Autodesk Fusion 360 part; units mm, degrees
(part 5 of 6)
  spline S167 degree 3 poles (6.8323, 73.9658) (7.1559, 73.6374) (7.8437, 72.9395) (8.0667, 71.9824) (8.1848, 71.4756) knots 0 0 0 0 0.135648 0.28832 0.28832 0.28832 0.28832
  line L106 (11.9153, 74.5713) -> (11.9153, 64.2002)
  line L107 (11.9153, 64.2002) -> (10.1575, 64.2002)
  line L108 (10.1575, 64.2002) -> (10.1575, 74.5713)
  line L109 (10.1575, 74.5713) -> (11.9153, 74.5713)
  line L110 (18.6047, 74.5713) -> (18.6047, 64.2002)
  line L111 (18.6047, 64.2002) -> (17.0227, 64.2002)
  line L112 (17.0227, 64.2002) -> (17.0227, 65.7724)
  spline S168 degree 3 poles (17.0227, 65.7724) (16.8465, 65.453) (16.5467, 64.9096) (16.0919, 64.4902) (15.9045, 64.3174) knots 0 0 0 0 0.1085 0.184546 0.184546 0.184546 0.184546
  spline S169 degree 3 poles (15.9045, 64.3174) (15.7296, 64.2148) (15.3808, 64.0103) (14.9776, 63.9806) (14.7766, 63.9658) knots 0 0 0 0 0.059943 0.119555 0.119555 0.119555 0.119555
  spline S170 degree 3 poles (14.7766, 63.9658) (14.4721, 63.9939) (13.8303, 64.053) (13.2663, 64.3671) (12.97, 64.5322) knots 0 0 0 0 0.090712 0.191197 0.191197 0.191197 0.191197
  line L113 (12.97, 64.5322) -> (13.5754, 66.1631)
  spline S171 degree 3 poles (13.5754, 66.1631) (13.7857, 66.052) (14.1903, 65.8384) (14.6457, 65.8004) (14.8645, 65.7822) knots 0 0 0 0 0.070499 0.135652 0.135652 0.135652 0.135652
  spline S172 degree 3 poles (14.8645, 65.7822) (15.0516, 65.7966) (15.4257, 65.8254) (15.7417, 66.0278) (15.8996, 66.1289) knots 0 0 0 0 0.05537 0.110689 0.110689 0.110689 0.110689
  spline S173 degree 3 poles (15.8996, 66.1289) (16.0426, 66.2586) (16.3376, 66.5264) (16.4803, 66.8988) (16.5539, 67.0908) knots 0 0 0 0 0.057074 0.117791 0.117791 0.117791 0.117791
  spline S174 degree 3 poles (16.5539, 67.0908) (16.6394, 67.4162) (16.8158, 68.0883) (16.8363, 68.7831) (16.8469, 69.1416) knots 0 0 0 0 0.100574 0.207758 0.207758 0.207758 0.207758
  line L114 (16.8469, 69.1416) -> (16.8469, 74.5713)
  line L115 (16.8469, 74.5713) -> (18.6047, 74.5713)
  line L116 (40.3918, 71.2314) -> (38.5754, 71.456)
  spline S175 degree 3 poles (38.5754, 71.456) (38.7423, 71.9516) (39.0652, 72.9106) (39.8082, 73.5957) (40.1672, 73.9267) knots 0 0 0 0 0.154068 0.298151 0.298151 0.298151 0.298151
  spline S176 degree 3 poles (40.1672, 73.9267) (40.5971, 74.1828) (41.5099, 74.7266) (42.5734, 74.7783) (43.136, 74.8056) knots 0 0 0 0 0.147834 0.313845 0.313845 0.313845 0.313845
  spline S177 degree 3 poles (43.136, 74.8056) (43.8438, 74.7587) (45.1975, 74.669) (46.2447, 73.8128) (46.7444, 73.4043) knots 0 0 0 0 0.206966 0.395783 0.395783 0.395783 0.395783
  spline S178 degree 3 poles (46.7444, 73.4043) (47.1326, 72.8627) (47.9713, 71.6927) (48.0403, 70.249) (48.0774, 69.4736) knots 0 0 0 0 0.195785 0.422974 0.422974 0.422974 0.422974
  spline S179 degree 3 poles (48.0774, 69.4736) (48.0408, 68.6725) (47.973, 67.1854) (47.1222, 65.9712) (46.7297, 65.4111) knots 0 0 0 0 0.234851 0.435929 0.435929 0.435929 0.435929
  spline S180 degree 3 poles (46.7297, 65.4111) (46.239, 64.9896) (45.2337, 64.1262) (43.9108, 64.0201) (43.2336, 63.9658) knots 0 0 0 0 0.188967 0.387114 0.387114 0.387114 0.387114
  spline S181 degree 3 poles (43.2336, 63.9658) (42.5767, 64.0198) (41.2894, 64.1256) (40.3132, 64.9688) (39.8352, 65.3818) knots 0 0 0 0 0.192252 0.37676 0.37676 0.37676 0.37676
  spline S182 degree 3 poles (39.8352, 65.3818) (39.4513, 65.931) (38.6184, 67.1223) (38.5524, 68.5803) (38.5168, 69.3662) knots 0 0 0 0 0.197018 0.427415 0.427415 0.427415 0.427415
  spline S183 degree 3 poles (38.5168, 69.3662) (38.5175, 69.4313) (38.5189, 69.5876) (38.5238, 69.7438) (38.5266, 69.8349) knots 0 0 0 0 0.019533 0.046886 0.046886 0.046886 0.046886
  line L117 (38.5266, 69.8349) -> (46.261, 69.8349)
  spline S184 degree 3 poles (46.261, 69.8349) (46.2102, 70.3557) (46.1165, 71.3165) (45.5525, 72.0954) (45.2942, 72.4521) knots 0 0 0 0 0.153651 0.283492 0.283492 0.283492 0.283492
  spline S185 degree 3 poles (45.2942, 72.4521) (44.9846, 72.717) (44.3597, 73.2517) (43.5399, 73.3239) (43.1262, 73.3603) knots 0 0 0 0 0.119065 0.24035 0.24035 0.24035 0.24035
  spline S186 degree 3 poles (43.1262, 73.3603) (42.8199, 73.3422) (42.2277, 73.3072) (41.7207, 73.0006) (41.4758, 72.8525) knots 0 0 0 0 0.090495 0.175003 0.175003 0.175003 0.175003
  spline S187 degree 3 poles (41.4758, 72.8525) (41.255, 72.6441) (40.7715, 72.1877) (40.5255, 71.5681) (40.3918, 71.2314) knots 0 0 0 0 0.090002 0.197114 0.197114 0.197114 0.197114
  line L118 (64.1711, 74.5713) -> (64.1711, 64.2002)
  line L119 (64.1711, 64.2002) -> (62.5891, 64.2002)
  line L120 (62.5891, 64.2002) -> (62.5891, 65.6748)
  spline S188 degree 3 poles (62.5891, 65.6748) (62.1608, 65.1763) (61.2915, 64.1647) (59.9625, 64.0328) (59.2883, 63.9658) knots 0 0 0 0 0.189553 0.384716 0.384716 0.384716 0.384716
  spline S189 degree 3 poles (59.2883, 63.9658) (58.9854, 63.9785) (58.3935, 64.0032) (57.8366, 64.2045) (57.5647, 64.3027) knots 0 0 0 0 0.090359 0.176544 0.176544 0.176544 0.176544
  spline S190 degree 3 poles (57.5647, 64.3027) (57.3239, 64.4173) (56.8712, 64.6327) (56.5421, 65.0099) (56.3879, 65.1865) knots 0 0 0 0 0.078991 0.148563 0.148563 0.148563 0.148563
  spline S191 degree 3 poles (56.3879, 65.1865) (56.2667, 65.3814) (56.0155, 65.785) (55.9005, 66.2466) (55.841, 66.4853) knots 0 0 0 0 0.068412 0.1417 0.1417 0.1417 0.1417
  spline S192 degree 3 poles (55.841, 66.4853) (55.8129, 66.7089) (55.7414, 67.276) (55.7426, 67.8478) (55.7434, 68.1943) knots 0 0 0 0 0.067537 0.171325 0.171325 0.171325 0.171325
  line L121 (55.7434, 68.1943) -> (55.7434, 74.5713)
  line L122 (55.7434, 74.5713) -> (57.5012, 74.5713)
  line L123 (57.5012, 74.5713) -> (57.5012, 68.2627)
  spline S193 degree 3 poles (57.5012, 68.2627) (57.5029, 67.9476) (57.5058, 67.4028) (57.6468, 66.8776) (57.7063, 66.6562) knots 0 0 0 0 0.094012 0.162533 0.162533 0.162533 0.162533
  spline S194 degree 3 poles (57.7063, 66.6562) (57.7895, 66.4868) (57.959, 66.1415) (58.2736, 65.9196) (58.4338, 65.8066) knots 0 0 0 0 0.055666 0.113464 0.113464 0.113464 0.113464
  spline S195 degree 3 poles (58.4338, 65.8066) (58.6195, 65.7141) (59.0052, 65.5219) (59.436, 65.5004) (59.6594, 65.4892) knots 0 0 0 0 0.061552 0.127824 0.127824 0.127824 0.127824
  spline S196 degree 3 poles (59.6594, 65.4892) (60.0196, 65.5177) (60.7327, 65.5742) (61.3114, 65.9942) (61.5979, 66.2021) knots 0 0 0 0 0.106122 0.210147 0.210147 0.210147 0.210147
  spline S197 degree 3 poles (61.5979, 66.2021) (61.8341, 66.5354) (62.4018, 67.3364) (62.4091, 68.3281) (62.4133, 68.9072) knots 0 0 0 0 0.120022 0.288496 0.288496 0.288496 0.288496
  line L124 (62.4133, 68.9072) -> (62.4133, 74.5713)
  line L125 (62.4133, 74.5713) -> (64.1711, 74.5713)
  line L126 (80, 80) -> (-25, 80)
  line L127 (-25, 80) -> (-25, 30)
  line L128 (-25, 30) -> (80, 30)
  line L129 (80, 30) -> (80, 80)
  line L130 (-9.6179, 71.2314) -> (-11.4343, 71.456)
  spline S198 degree 3 poles (-11.4343, 71.456) (-11.2675, 71.9516) (-10.9445, 72.9106) (-10.2016, 73.5957) (-9.8425, 73.9267) knots 0 0 0 0 0.154068 0.298151 0.298151 0.298151 0.298151
  spline S199 degree 3 poles (-9.8425, 73.9267) (-9.4126, 74.1828) (-8.4999, 74.7266) (-7.4364, 74.7783) (-6.8738, 74.8056) knots 0 0 0 0 0.147834 0.313845 0.313845 0.313845 0.313845
  spline S200 degree 3 poles (-6.8738, 74.8056) (-6.1659, 74.7587) (-4.8123, 74.669) (-3.765, 73.8128) (-3.2654, 73.4043) knots 0 0 0 0 0.206966 0.395783 0.395783 0.395783 0.395783
  spline S201 degree 3 poles (-3.2654, 73.4043) (-2.8772, 72.8627) (-2.0385, 71.6927) (-1.9695, 70.249) (-1.9324, 69.4736) knots 0 0 0 0 0.195785 0.422974 0.422974 0.422974 0.422974
  spline S202 degree 3 poles (-1.9324, 69.4736) (-1.9689, 68.6725) (-2.0368, 67.1854) (-2.8876, 65.9712) (-3.28, 65.4111) knots 0 0 0 0 0.234851 0.435929 0.435929 0.435929 0.435929
  spline S203 degree 3 poles (-3.28, 65.4111) (-3.7708, 64.9896) (-4.776, 64.1262) (-6.099, 64.0201) (-6.7761, 63.9658) knots 0 0 0 0 0.188967 0.387114 0.387114 0.387114 0.387114
  spline S204 degree 3 poles (-6.7761, 63.9658) (-7.433, 64.0198) (-8.7203, 64.1256) (-9.6965, 64.9688) (-10.1746, 65.3818) knots 0 0 0 0 0.192252 0.37676 0.37676 0.37676 0.37676
  spline S205 degree 3 poles (-10.1746, 65.3818) (-10.5585, 65.931) (-11.3913, 67.1223) (-11.4573, 68.5803) (-11.4929, 69.3662) knots 0 0 0 0 0.197018 0.427415 0.427415 0.427415 0.427415
  spline S206 degree 3 poles (-11.4929, 69.3662) (-11.4923, 69.4313) (-11.4908, 69.5876) (-11.486, 69.7438) (-11.4832, 69.8349) knots 0 0 0 0 0.019533 0.046886 0.046886 0.046886 0.046886
  line L131 (-11.4832, 69.8349) -> (-3.7488, 69.8349)
  spline S207 degree 3 poles (-3.7488, 69.8349) (-3.7996, 70.3557) (-3.8933, 71.3165) (-4.4573, 72.0954) (-4.7156, 72.4521) knots 0 0 0 0 0.153651 0.283492 0.283492 0.283492 0.283492
  spline S208 degree 3 poles (-4.7156, 72.4521) (-5.0252, 72.717) (-5.6501, 73.2517) (-6.4699, 73.3239) (-6.8836, 73.3603) knots 0 0 0 0 0.119065 0.24035 0.24035 0.24035 0.24035
  spline S209 degree 3 poles (-6.8836, 73.3603) (-7.1898, 73.3422) (-7.7821, 73.3072) (-8.2891, 73.0006) (-8.534, 72.8525) knots 0 0 0 0 0.090495 0.175003 0.175003 0.175003 0.175003
  spline S210 degree 3 poles (-8.534, 72.8525) (-8.7547, 72.6441) (-9.2382, 72.1877) (-9.4842, 71.5681) (-9.6179, 71.2314) knots 0 0 0 0 0.090002 0.197114 0.197114 0.197114 0.197114
  line L132 (36.3879, 74.5713) -> (36.3879, 64.2002)
  line L133 (36.3879, 64.2002) -> (34.8059, 64.2002)
  line L134 (34.8059, 64.2002) -> (34.8059, 65.7724)
  spline S211 degree 3 poles (34.8059, 65.7724) (34.6297, 65.453) (34.3299, 64.9096) (33.8751, 64.4902) (33.6877, 64.3174) knots 0 0 0 0 0.1085 0.184546 0.184546 0.184546 0.184546
  spline S212 degree 3 poles (33.6877, 64.3174) (33.5128, 64.2148) (33.164, 64.0103) (32.7608, 63.9806) (32.5598, 63.9658) knots 0 0 0 0 0.059943 0.119555 0.119555 0.119555 0.119555
  spline S213 degree 3 poles (32.5598, 63.9658) (32.2553, 63.9939) (31.6135, 64.053) (31.0495, 64.3671) (30.7532, 64.5322) knots 0 0 0 0 0.090712 0.191197 0.191197 0.191197 0.191197
  line L135 (30.7532, 64.5322) -> (31.3586, 66.1631)
  spline S214 degree 3 poles (31.3586, 66.1631) (31.5689, 66.052) (31.9735, 65.8384) (32.4289, 65.8004) (32.6477, 65.7822) knots 0 0 0 0 0.070499 0.135652 0.135652 0.135652 0.135652
  spline S215 degree 3 poles (32.6477, 65.7822) (32.8348, 65.7966) (33.2089, 65.8254) (33.5249, 66.0278) (33.6828, 66.1289) knots 0 0 0 0 0.05537 0.110689 0.110689 0.110689 0.110689
  spline S216 degree 3 poles (33.6828, 66.1289) (33.8258, 66.2586) (34.1208, 66.5264) (34.2635, 66.8988) (34.3371, 67.0908) knots 0 0 0 0 0.057074 0.117791 0.117791 0.117791 0.117791
  spline S217 degree 3 poles (34.3371, 67.0908) (34.4226, 67.4162) (34.599, 68.0883) (34.6195, 68.7831) (34.6301, 69.1416) knots 0 0 0 0 0.100574 0.207758 0.207758 0.207758 0.207758
  line L136 (34.6301, 69.1416) -> (34.6301, 74.5713)
  line L137 (34.6301, 74.5713) -> (36.3879, 74.5713)
  line L138 (49.2102, 72.999) -> (48.9563, 74.5517)
  spline S218 degree 3 poles (48.9563, 74.5517) (49.1899, 74.5972) (49.6288, 74.6827) (50.0755, 74.6999) (50.2844, 74.708) knots 0 0 0 0 0.071282 0.133904 0.133904 0.133904 0.133904
  spline S219 degree 3 poles (50.2844, 74.708) (50.5719, 74.7024) (51.0867, 74.6925) (51.5599, 74.4932) (51.7688, 74.4052) knots 0 0 0 0 0.085297 0.152712 0.152712 0.152712 0.152712
  spline S220 degree 3 poles (51.7688, 74.4052) (51.9303, 74.2993) (52.2429, 74.0941) (52.4236, 73.7673) (52.511, 73.6093) knots 0 0 0 0 0.056968 0.110293 0.110293 0.110293 0.110293
  spline S221 degree 3 poles (52.511, 73.6093) (52.5727, 73.3552) (52.738, 72.6752) (52.7305, 71.9736) (52.7258, 71.5341) knots 0 0 0 0 0.078216 0.209307 0.209307 0.209307 0.209307
  line L139 (52.7258, 71.5341) -> (52.7258, 65.5674)
  line L140 (52.7258, 65.5674) -> (54.0149, 65.5674)
  line L141 (54.0149, 65.5674) -> (54.0149, 64.2002)
  line L142 (54.0149, 64.2002) -> (52.7258, 64.2002)
  line L143 (52.7258, 64.2002) -> (52.7258, 61.6318)
  line L144 (52.7258, 61.6318) -> (50.9778, 60.5771)
  line L145 (50.9778, 60.5771) -> (50.9778, 64.2002)
  line L146 (50.9778, 64.2002) -> (49.2102, 64.2002)
  line L147 (49.2102, 64.2002) -> (49.2102, 65.5674)
  line L148 (49.2102, 65.5674) -> (50.9778, 65.5674)
  line L149 (50.9778, 65.5674) -> (50.9778, 71.6318)
  spline S222 degree 3 poles (50.9778, 71.6318) (50.9804, 71.8389) (50.9844, 72.1653) (50.9116, 72.4826) (50.885, 72.5986) knots 0 0 0 0 0.061811 0.09741 0.09741 0.09741 0.09741
  spline S223 degree 3 poles (50.885, 72.5986) (50.8488, 72.6668) (50.7753, 72.805) (50.6472, 72.8949) (50.5823, 72.9404) knots 0 0 0 0 0.022826 0.046239 0.046239 0.046239 0.046239
  spline S224 degree 3 poles (50.5823, 72.9404) (50.4984, 72.9773) (50.3077, 73.0612) (50.0987, 73.0651) (49.9817, 73.0674) knots 0 0 0 0 0.027232 0.061923 0.061923 0.061923 0.061923
  spline S225 degree 3 poles (49.9817, 73.0674) (49.8684, 73.0633) (49.6101, 73.0542) (49.354, 73.0188) (49.2102, 72.999) knots 0 0 0 0 0.033979 0.077495 0.077495 0.077495 0.077495
  line L150 (77.2473, 74.5713) -> (77.2473, 60.2549)
  line L151 (77.2473, 60.2549) -> (66.8957, 60.2549)
  line L152 (66.8957, 60.2549) -> (66.8957, 61.9443)
  line L153 (66.8957, 61.9443) -> (75.3528, 61.9443)
  line L154 (75.3528, 61.9443) -> (75.3528, 66.3291)
  line L155 (75.3528, 66.3291) -> (67.4328, 66.3291)
  line L156 (67.4328, 66.3291) -> (67.4328, 68.0088)
  line L157 (67.4328, 68.0088) -> (75.3528, 68.0088)
  line L158 (75.3528, 68.0088) -> (75.3528, 72.8818)
  line L159 (75.3528, 72.8818) -> (66.5637, 72.8818)
  line L160 (66.5637, 72.8818) -> (66.5637, 74.5713)
  line L161 (66.5637, 74.5713) -> (77.2473, 74.5713)
  line L162 (65.1829, 55.7007) -> (65.1829, 47.9224)
  line L163 (65.1829, 47.9224) -> (63.9963, 47.9224)
  line L164 (63.9963, 47.9224) -> (63.9963, 49.0283)
  spline S226 degree 3 poles (63.9963, 49.0283) (63.6751, 48.6545) (63.0232, 47.8958) (62.0264, 47.7968) (61.5208, 47.7466) knots 0 0 0 0 0.142165 0.288537 0.288537 0.288537 0.288537
  spline S227 degree 3 poles (61.5208, 47.7466) (61.2936, 47.7561) (60.8496, 47.7746) (60.4319, 47.9256) (60.228, 47.9993) knots 0 0 0 0 0.067769 0.132408 0.132408 0.132408 0.132408
  spline S228 degree 3 poles (60.228, 47.9993) (60.0475, 48.0852) (59.7079, 48.2468) (59.4611, 48.5296) (59.3455, 48.6621) knots 0 0 0 0 0.059243 0.111422 0.111422 0.111422 0.111422
  spline S229 degree 3 poles (59.3455, 48.6621) (59.2545, 48.8083) (59.0662, 49.111) (58.9799, 49.4572) (58.9353, 49.6362) knots 0 0 0 0 0.051309 0.106275 0.106275 0.106275 0.106275
  spline S230 degree 3 poles (58.9353, 49.6362) (58.9142, 49.8039) (58.8606, 50.2292) (58.8615, 50.6581) (58.8621, 50.918) knots 0 0 0 0 0.050653 0.128494 0.128494 0.128494 0.128494
  line L165 (58.8621, 50.918) -> (58.8621, 55.7007)
  line L166 (58.8621, 55.7007) -> (60.1804, 55.7007)
  line L167 (60.1804, 55.7007) -> (60.1804, 50.9692)
  spline S231 degree 3 poles (60.1804, 50.9692) (60.1817, 50.7329) (60.1839, 50.3244) (60.2896, 49.9305) (60.3342, 49.7644) knots 0 0 0 0 0.070509 0.1219 0.1219 0.1219 0.1219
  spline S232 degree 3 poles (60.3342, 49.7644) (60.3966, 49.6373) (60.5238, 49.3784) (60.7597, 49.212) (60.8799, 49.1272) knots 0 0 0 0 0.04175 0.085098 0.085098 0.085098 0.085098
  spline S233 degree 3 poles (60.8799, 49.1272) (61.0192, 49.0578) (61.3084, 48.9137) (61.6316, 48.8975) (61.7991, 48.8892) knots 0 0 0 0 0.046164 0.095868 0.095868 0.095868 0.095868
  spline S234 degree 3 poles (61.7991, 48.8892) (62.0692, 48.9105) (62.6041, 48.9529) (63.0381, 49.2679) (63.2529, 49.4238) knots 0 0 0 0 0.079591 0.15761 0.15761 0.15761 0.15761
  spline S235 degree 3 poles (63.2529, 49.4238) (63.4301, 49.6738) (63.8559, 50.2745) (63.8613, 51.0183) (63.8645, 51.4526) knots 0 0 0 0 0.090016 0.216372 0.216372 0.216372 0.216372
  line L168 (63.8645, 51.4526) -> (63.8645, 55.7007)
  line L169 (63.8645, 55.7007) -> (65.1829, 55.7007)
  line L170 (47.3484, 53.1958) -> (45.9861, 53.3643)
  spline S236 degree 3 poles (45.9861, 53.3643) (46.1113, 53.7359) (46.3535, 54.4552) (46.9107, 54.969) (47.1799, 55.2173) knots 0 0 0 0 0.115551 0.223613 0.223613 0.223613 0.223613
  spline S237 degree 3 poles (47.1799, 55.2173) (47.5024, 55.4094) (48.1869, 55.8172) (48.9846, 55.8559) (49.4065, 55.8765) knots 0 0 0 0 0.110875 0.235384 0.235384 0.235384 0.235384
  spline S238 degree 3 poles (49.4065, 55.8765) (49.9374, 55.8413) (50.9526, 55.774) (51.7381, 55.1318) (52.1128, 54.8254) knots 0 0 0 0 0.155225 0.296837 0.296837 0.296837 0.296837
  spline S239 degree 3 poles (52.1128, 54.8254) (52.404, 54.4193) (53.033, 53.5417) (53.0848, 52.459) (53.1126, 51.8774) knots 0 0 0 0 0.146839 0.31723 0.31723 0.31723 0.31723
  spline S240 degree 3 poles (53.1126, 51.8774) (53.0851, 51.2766) (53.0342, 50.1613) (52.3961, 49.2506) (52.1018, 48.8306) knots 0 0 0 0 0.176138 0.326947 0.326947 0.326947 0.326947
  spline S241 degree 3 poles (52.1018, 48.8306) (51.7338, 48.5145) (50.9798, 47.8669) (49.9876, 47.7873) (49.4797, 47.7466) knots 0 0 0 0 0.141726 0.290335 0.290335 0.290335 0.290335
  spline S242 degree 3 poles (49.4797, 47.7466) (48.9871, 47.7871) (48.0216, 47.8664) (47.2895, 48.4989) (46.9309, 48.8086) knots 0 0 0 0 0.144189 0.28257 0.28257 0.28257 0.28257
  spline S243 degree 3 poles (46.9309, 48.8086) (46.643, 49.2205) (46.0184, 50.114) (45.9688, 51.2074) (45.9421, 51.7969) knots 0 0 0 0 0.147764 0.320562 0.320562 0.320562 0.320562
  spline S244 degree 3 poles (45.9421, 51.7969) (45.9426, 51.8457) (45.9437, 51.9629) (45.9474, 52.0801) (45.9495, 52.1484) knots 0 0 0 0 0.01465 0.035165 0.035165 0.035165 0.035165
  line L171 (45.9495, 52.1484) -> (51.7503, 52.1484)
  spline S245 degree 3 poles (51.7503, 52.1484) (51.7122, 52.539) (51.6419, 53.2596) (51.2189, 53.8438) (51.0252, 54.1113) knots 0 0 0 0 0.115238 0.212619 0.212619 0.212619 0.212619
  spline S246 degree 3 poles (51.0252, 54.1113) (50.793, 54.31) (50.3243, 54.711) (49.7094, 54.7652) (49.3992, 54.7925) knots 0 0 0 0 0.089299 0.180262 0.180262 0.180262 0.180262
  spline S247 degree 3 poles (49.3992, 54.7925) (49.1695, 54.7789) (48.7253, 54.7526) (48.345, 54.5227) (48.1614, 54.4116) knots 0 0 0 0 0.067871 0.131252 0.131252 0.131252 0.131252
  spline S248 degree 3 poles (48.1614, 54.4116) (47.9958, 54.2553) (47.6332, 53.913) (47.4487, 53.4483) (47.3484, 53.1958) knots 0 0 0 0 0.067501 0.147835 0.147835 0.147835 0.147835
  line L172 (31.0081, 55.7007) -> (31.0081, 47.9224)
  line L173 (31.0081, 47.9224) -> (29.8215, 47.9224)
  line L174 (29.8215, 47.9224) -> (29.8215, 49.1016)
  spline S249 degree 3 poles (29.8215, 49.1016) (29.6894, 48.862) (29.4646, 48.4545) (29.1235, 48.1399) (28.9829, 48.0103) knots 0 0 0 0 0.081375 0.138409 0.138409 0.138409 0.138409
  spline S250 degree 3 poles (28.9829, 48.0103) (28.8518, 47.9333) (28.5902, 47.78) (28.2878, 47.7577) (28.137, 47.7466) knots 0 0 0 0 0.044958 0.089666 0.089666 0.089666 0.089666
  spline S251 degree 3 poles (28.137, 47.7466) (27.9086, 47.7676) (27.4272, 47.812) (27.0043, 48.0476) (26.782, 48.1714) knots 0 0 0 0 0.068034 0.143398 0.143398 0.143398 0.143398
  line L175 (26.782, 48.1714) -> (27.2361, 49.3945)
  spline S252 degree 3 poles (27.2361, 49.3945) (27.3938, 49.3113) (27.6972, 49.151) (28.0388, 49.1226) (28.2029, 49.1089) knots 0 0 0 0 0.052874 0.101739 0.101739 0.101739 0.101739
  spline S253 degree 3 poles (28.2029, 49.1089) (28.3432, 49.1197) (28.6238, 49.1413) (28.8608, 49.2931) (28.9793, 49.3689) knots 0 0 0 0 0.041528 0.083017 0.083017 0.083017 0.083017
  spline S254 degree 3 poles (28.9793, 49.3689) (29.0865, 49.4662) (29.3077, 49.667) (29.4148, 49.9464) (29.47, 50.0903) knots 0 0 0 0 0.042806 0.088343 0.088343 0.088343 0.088343
  spline S255 degree 3 poles (29.47, 50.0903) (29.534, 50.3344) (29.6664, 50.8385) (29.6818, 51.3596) (29.6897, 51.6284) knots 0 0 0 0 0.075431 0.155819 0.155819 0.155819 0.155819
  line L176 (29.6897, 51.6284) -> (29.6897, 55.7007)
  line L177 (29.6897, 55.7007) -> (31.0081, 55.7007)
  line L178 (25.991, 55.7007) -> (25.991, 47.9224)
  line L179 (25.991, 47.9224) -> (24.6726, 47.9224)
  line L180 (24.6726, 47.9224) -> (24.6726, 55.7007)
  line L181 (24.6726, 55.7007) -> (25.991, 55.7007)
  line L182 (23.1931, 53.3789) -> (21.8894, 53.1738)
  spline S256 degree 3 poles (21.8894, 53.1738) (21.8413, 53.4156) (21.75, 53.8747) (21.4295, 54.2143) (21.2778, 54.375) knots 0 0 0 0 0.072267 0.137238 0.137238 0.137238 0.137238
  spline S257 degree 3 poles (21.2778, 54.375) (21.0827, 54.4965) (20.6552, 54.7628) (20.1499, 54.782) (19.8753, 54.7925) knots 0 0 0 0 0.067812 0.148597 0.148597 0.148597 0.148597
  spline S258 degree 3 poles (19.8753, 54.7925) (19.6043, 54.7862) (19.1216, 54.7751) (18.7087, 54.5301) (18.5276, 54.4226) knots 0 0 0 0 0.07964 0.141834 0.141834 0.141834 0.141834
  spline S259 degree 3 poles (18.5276, 54.4226) (18.3995, 54.2977) (18.1534, 54.0576) (18.1093, 53.7177) (18.0881, 53.5547) knots 0 0 0 0 0.051978 0.099855 0.099855 0.099855 0.099855
  spline S260 degree 3 poles (18.0881, 53.5547) (18.1051, 53.4132) (18.1394, 53.1267) (18.3631, 52.944) (18.4763, 52.8516) knots 0 0 0 0 0.04108 0.083169 0.083169 0.083169 0.083169
  spline S261 degree 3 poles (18.4763, 52.8516) (18.6325, 52.7814) (19.0657, 52.5869) (19.5282, 52.4758) (19.824, 52.4048) knots 0 0 0 0 0.051284 0.142232 0.142232 0.142232 0.142232
  spline S262 degree 3 poles (19.824, 52.4048) (20.2366, 52.3014) (20.9198, 52.1303) (21.575, 51.8731) (21.8345, 51.7712) knots 0 0 0 0 0.127433 0.210981 0.210981 0.210981 0.210981
  spline S263 degree 3 poles (21.8345, 51.7712) (22.0084, 51.6761) (22.346, 51.4914) (22.5737, 51.1817) (22.6841, 51.0315) knots 0 0 0 0 0.058662 0.113875 0.113875 0.113875 0.113875
  spline S264 degree 3 poles (22.6841, 51.0315) (22.7685, 50.8691) (22.9386, 50.5418) (22.9617, 50.1734) (22.9734, 49.9878) knots 0 0 0 0 0.054242 0.109375 0.109375 0.109375 0.109375
  spline S265 degree 3 poles (22.9734, 49.9878) (22.9638, 49.8183) (22.9449, 49.4823) (22.8048, 49.1763) (22.7354, 49.0247) knots 0 0 0 0 0.050432 0.099993 0.099993 0.099993 0.099993
  spline S266 degree 3 poles (22.7354, 49.0247) (22.6488, 48.8832) (22.4756, 48.6001) (22.2167, 48.3924) (22.0872, 48.2886) knots 0 0 0 0 0.049345 0.098743 0.098743 0.098743 0.098743
  spline S267 degree 3 poles (22.0872, 48.2886) (21.9683, 48.2138) (21.706, 48.0488) (21.4103, 47.9552) (21.2485, 47.904) knots 0 0 0 0 0.04196 0.092591 0.092591 0.092591 0.092591
  spline S268 degree 3 poles (21.2485, 47.904) (21.0661, 47.8581) (20.6922, 47.7641) (20.3069, 47.7525) (20.1096, 47.7466) knots 0 0 0 0 0.056276 0.115276 0.115276 0.115276 0.115276
  spline S269 degree 3 poles (20.1096, 47.7466) (19.8208, 47.755) (19.2727, 47.7709) (18.7494, 47.9334) (18.502, 48.0103) knots 0 0 0 0 0.08622 0.163589 0.163589 0.163589 0.163589
  spline S270 degree 3 poles (18.502, 48.0103) (18.2913, 48.0995) (17.8993, 48.2656) (17.6128, 48.5793) (17.4802, 48.7244) knots 0 0 0 0 0.067685 0.125961 0.125961 0.125961 0.125961
  spline S271 degree 3 poles (17.4802, 48.7244) (17.3776, 48.896) (17.1541, 49.2697) (17.0711, 49.6978) (17.0261, 49.9292) knots 0 0 0 0 0.059547 0.129628 0.129628 0.129628 0.129628
  line L183 (17.0261, 49.9292) -> (18.3152, 50.105)
  spline S272 degree 3 poles (18.3152, 50.105) (18.3559, 49.9178) (18.4349, 49.5552) (18.6973, 49.2939) (18.8242, 49.1675) knots 0 0 0 0 0.056141 0.108715 0.108715 0.108715 0.108715
  spline S273 degree 3 poles (18.8242, 49.1675) (18.9894, 49.0694) (19.3548, 48.8527) (19.781, 48.8384) (20.0144, 48.8306) knots 0 0 0 0 0.056748 0.125473 0.125473 0.125473 0.125473
  spline S274 degree 3 poles (20.0144, 48.8306) (20.2797, 48.8327) (20.7368, 48.8364) (21.1412, 49.0438) (21.3108, 49.1309) knots 0 0 0 0 0.078181 0.134683 0.134683 0.134683 0.134683
  spline S275 degree 3 poles (21.3108, 49.1309) (21.4239, 49.2309) (21.6378, 49.4202) (21.6794, 49.7014) (21.699, 49.834) knots 0 0 0 0 0.043702 0.082651 0.082651 0.082651 0.082651
  spline S276 degree 3 poles (21.699, 49.834) (21.6921, 49.9175) (21.6784, 50.0852) (21.5848, 50.2251) (21.5379, 50.2954) knots 0 0 0 0 0.024684 0.0496 0.0496 0.0496 0.0496
  spline S277 degree 3 poles (21.5379, 50.2954) (21.4722, 50.3648) (21.3286, 50.5167) (21.1367, 50.6011) (21.0325, 50.647) knots 0 0 0 0 0.02837 0.062115 0.062115 0.062115 0.062115
  spline S278 degree 3 poles (21.0325, 50.647) (20.9027, 50.6879) (20.5172, 50.8093) (20.1268, 50.9143) (19.8679, 50.9839) knots 0 0 0 0 0.040831 0.121242 0.121242 0.121242 0.121242
  spline S279 degree 3 poles (19.8679, 50.9839) (19.4697, 51.0896) (18.8099, 51.2649) (18.1698, 51.5016) (17.916, 51.5955) knots 0 0 0 0 0.123506 0.204645 0.204645 0.204645 0.204645
  spline S280 degree 3 poles (17.916, 51.5955) (17.7429, 51.682) (17.4043, 51.8513) (17.165, 52.1444) (17.0481, 52.2876) knots 0 0 0 0 0.057342 0.11214 0.11214 0.11214 0.11214
  spline S281 degree 3 poles (17.0481, 52.2876) (16.9563, 52.4535) (16.7625, 52.8039) (16.7433, 53.2046) (16.7332, 53.4155) knots 0 0 0 0 0.056117 0.118505 0.118505 0.118505 0.118505
  spline S282 degree 3 poles (16.7332, 53.4155) (16.7501, 53.6335) (16.7846, 54.0761) (17.0055, 54.4614) (17.1177, 54.657) knots 0 0 0 0 0.064713 0.13142 0.13142 0.13142 0.13142
  spline S283 degree 3 poles (17.1177, 54.657) (17.2639, 54.8417) (17.5664, 55.2241) (18.0021, 55.4441) (18.2273, 55.5579) knots 0 0 0 0 0.0698 0.14446 0.14446 0.14446 0.14446
  spline S284 degree 3 poles (18.2273, 55.5579) (18.4822, 55.6507) (19.0119, 55.8437) (19.5756, 55.8653) (19.8679, 55.8765) knots 0 0 0 0 0.080881 0.168038 0.168038 0.168038 0.168038
  spline S285 degree 3 poles (19.8679, 55.8765) (20.3248, 55.8636) (21.1496, 55.8403) (21.8612, 55.4297) (22.1787, 55.2466) knots 0 0 0 0 0.1345 0.242846 0.242846 0.242846 0.242846
  spline S286 degree 3 poles (22.1787, 55.2466) (22.4214, 55.0003) (22.9373, 54.4768) (23.1046, 53.759) (23.1931, 53.3789) knots 0 0 0 0 0.101736 0.21624 0.21624 0.21624 0.21624
  line L184 (25.991, 46.4795) -> (25.991, 44.9634)
  line L185 (25.991, 44.9634) -> (24.6726, 44.9634)
  line L186 (24.6726, 44.9634) -> (24.6726, 46.4795)
  line L187 (24.6726, 46.4795) -> (25.991, 46.4795)
  line L188 (39.3357, 58.6816) -> (39.3357, 47.9224)
  line L189 (39.3357, 47.9224) -> (38.1345, 47.9224)
  line L190 (38.1345, 47.9224) -> (38.1345, 48.9331)
  spline S287 degree 3 poles (38.1345, 48.9331) (37.9928, 48.7502) (37.7217, 48.4005) (37.3516, 48.1586) (37.1751, 48.0432) knots 0 0 0 0 0.068849 0.131677 0.131677 0.131677 0.131677
  spline S288 degree 3 poles (37.1751, 48.0432) (36.9808, 47.9568) (36.5687, 47.7734) (36.1173, 47.7558) (35.8787, 47.7466) knots 0 0 0 0 0.063189 0.134074 0.134074 0.134074 0.134074
  spline S289 degree 3 poles (35.8787, 47.7466) (35.5593, 47.766) (34.9341, 47.8041) (34.388, 48.1098) (34.1209, 48.2593) knots 0 0 0 0 0.094622 0.185218 0.185218 0.185218 0.185218
  spline S290 degree 3 poles (34.1209, 48.2593) (33.881, 48.4515) (33.3885, 48.8462) (33.1125, 49.4144) (32.971, 49.7058) knots 0 0 0 0 0.091026 0.186859 0.186859 0.186859 0.186859
  spline S291 degree 3 poles (32.971, 49.7058) (32.8578, 50.0289) (32.6256, 50.6916) (32.5973, 51.3934) (32.5828, 51.7529) knots 0 0 0 0 0.102108 0.20939 0.20939 0.20939 0.20939
  spline S292 degree 3 poles (32.5828, 51.7529) (32.5981, 52.1352) (32.6277, 52.8747) (32.8863, 53.5678) (33.0112, 53.9026) knots 0 0 0 0 0.113938 0.220434 0.220434 0.220434 0.220434
  spline S293 degree 3 poles (33.0112, 53.9026) (33.167, 54.2005) (33.4717, 54.7833) (33.9988, 55.1757) (34.2564, 55.3674) knots 0 0 0 0 0.099433 0.194467 0.194467 0.194467 0.194467
  spline S294 degree 3 poles (34.2564, 55.3674) (34.5294, 55.5159) (35.066, 55.8077) (35.6748, 55.8538) (35.9739, 55.8765) knots 0 0 0 0 0.09206 0.180958 0.180958 0.180958 0.180958
  spline S295 degree 3 poles (35.9739, 55.8765) (36.1854, 55.8662) (36.5971, 55.8462) (36.9737, 55.6793) (37.1567, 55.5981) knots 0 0 0 0 0.062916 0.122451 0.122451 0.122451 0.122451
  spline S296 degree 3 poles (37.1567, 55.5981) (37.3222, 55.501) (37.6455, 55.311) (37.8953, 55.0315) (38.0173, 54.895) knots 0 0 0 0 0.057158 0.111733 0.111733 0.111733 0.111733
  line L191 (38.0173, 54.895) -> (38.0173, 58.6816)
  line L192 (38.0173, 58.6816) -> (39.3357, 58.6816)
  line L193 (31.9125, 39.2233) -> (31.0043, 39.3356)
  spline S297 degree 3 poles (31.0043, 39.3356) (31.0877, 39.5834) (31.2492, 40.0629) (31.6207, 40.4055) (31.8002, 40.571) knots 0 0 0 0 0.077034 0.149075 0.149075 0.149075 0.149075
  spline S298 degree 3 poles (31.8002, 40.571) (32.0151, 40.699) (32.4715, 40.9709) (33.0033, 40.9968) (33.2845, 41.0104) knots 0 0 0 0 0.073917 0.156923 0.156923 0.156923 0.156923
  spline S299 degree 3 poles (33.2845, 41.0104) (33.6385, 40.987) (34.3153, 40.9421) (34.8389, 40.514) (35.0887, 40.3097) knots 0 0 0 0 0.103483 0.197891 0.197891 0.197891 0.197891
  spline S300 degree 3 poles (35.0887, 40.3097) (35.2829, 40.039) (35.7022, 39.454) (35.7367, 38.7321) (35.7552, 38.3444) knots 0 0 0 0 0.097893 0.211487 0.211487 0.211487 0.211487
  spline S301 degree 3 poles (35.7552, 38.3444) (35.737, 37.9438) (35.703, 37.2003) (35.2776, 36.5932) (35.0814, 36.3132) knots 0 0 0 0 0.117426 0.217964 0.217964 0.217964 0.217964
  spline S302 degree 3 poles (35.0814, 36.3132) (34.8361, 36.1024) (34.3334, 35.6707) (33.6719, 35.6177) (33.3334, 35.5905) knots 0 0 0 0 0.094484 0.193557 0.193557 0.193557 0.193557
  spline S303 degree 3 poles (33.3334, 35.5905) (33.0049, 35.6175) (32.3613, 35.6704) (31.8732, 36.092) (31.6342, 36.2985) knots 0 0 0 0 0.096126 0.18838 0.18838 0.18838 0.18838
  spline S304 degree 3 poles (31.6342, 36.2985) (31.4422, 36.5731) (31.0258, 37.1688) (30.9928, 37.8977) (30.975, 38.2907) knots 0 0 0 0 0.098509 0.213708 0.213708 0.213708 0.213708
  spline S305 degree 3 poles (30.975, 38.2907) (30.9753, 38.3233) (30.976, 38.4014) (30.9784, 38.4795) (30.9799, 38.5251) knots 0 0 0 0 0.009766 0.023443 0.023443 0.023443 0.023443
  line L194 (30.9799, 38.5251) -> (34.847, 38.5251)
  spline S306 degree 3 poles (34.847, 38.5251) (34.8216, 38.7854) (34.7748, 39.2658) (34.4928, 39.6553) (34.3636, 39.8337) knots 0 0 0 0 0.076825 0.141746 0.141746 0.141746 0.141746
  spline S307 degree 3 poles (34.3636, 39.8337) (34.2089, 39.9661) (33.8964, 40.2335) (33.4865, 40.2696) (33.2797, 40.2878) knots 0 0 0 0 0.059532 0.120175 0.120175 0.120175 0.120175
  spline S308 degree 3 poles (33.2797, 40.2878) (33.1265, 40.2787) (32.8304, 40.2612) (32.5769, 40.1079) (32.4545, 40.0339) knots 0 0 0 0 0.045247 0.087501 0.087501 0.087501 0.087501
  spline S309 degree 3 poles (32.4545, 40.0339) (32.3441, 39.9297) (32.1023, 39.7015) (31.9793, 39.3917) (31.9125, 39.2233) knots 0 0 0 0 0.045001 0.098557 0.098557 0.098557 0.098557
  line L195 (54.9154, 40.8932) -> (54.9154, 35.7077)
  line L196 (54.9154, 35.7077) -> (54.1244, 35.7077)
  line L197 (54.1244, 35.7077) -> (54.1244, 36.4938)
  spline S310 degree 3 poles (54.1244, 36.4938) (54.0363, 36.3341) (53.8864, 36.0624) (53.659, 35.8527) (53.5653, 35.7663) knots 0 0 0 0 0.05425 0.092273 0.092273 0.092273 0.092273
  spline S311 degree 3 poles (53.5653, 35.7663) (53.4779, 35.715) (53.3035, 35.6128) (53.1019, 35.5979) (53.0013, 35.5905) knots 0 0 0 0 0.029972 0.059777 0.059777 0.059777 0.059777
  spline S312 degree 3 poles (53.0013, 35.5905) (52.8491, 35.6045) (52.5282, 35.6341) (52.2462, 35.7912) (52.098, 35.8737) knots 0 0 0 0 0.045356 0.095599 0.095599 0.095599 0.095599
  line L198 (52.098, 35.8737) -> (52.4008, 36.6891)
  spline S313 degree 3 poles (52.4008, 36.6891) (52.5059, 36.6336) (52.7082, 36.5268) (52.9359, 36.5078) (53.0453, 36.4987) knots 0 0 0 0 0.03525 0.067826 0.067826 0.067826 0.067826
  spline S314 degree 3 poles (53.0453, 36.4987) (53.1389, 36.5059) (53.3259, 36.5203) (53.4839, 36.6215) (53.5629, 36.672) knots 0 0 0 0 0.027685 0.055345 0.055345 0.055345 0.055345
  spline S315 degree 3 poles (53.5629, 36.672) (53.6343, 36.7369) (53.7818, 36.8708) (53.8532, 37.057) (53.89, 37.153) knots 0 0 0 0 0.028537 0.058895 0.058895 0.058895 0.058895
  spline S316 degree 3 poles (53.89, 37.153) (53.9327, 37.3157) (54.021, 37.6518) (54.0312, 37.9992) (54.0365, 38.1784) knots 0 0 0 0 0.050287 0.103879 0.103879 0.103879 0.103879
  line L199 (54.0365, 38.1784) -> (54.0365, 40.8932)
  line L200 (54.0365, 40.8932) -> (54.9154, 40.8932)
  line L201 (61.3265, 40.1071) -> (61.1996, 40.8835)
  spline S317 degree 3 poles (61.1996, 40.8835) (61.3164, 40.9062) (61.5358, 40.949) (61.7592, 40.9576) (61.8636, 40.9616) knots 0 0 0 0 0.035641 0.066952 0.066952 0.066952 0.066952
  spline S318 degree 3 poles (61.8636, 40.9616) (62.0074, 40.9588) (62.2648, 40.9539) (62.5014, 40.8542) (62.6058, 40.8102) knots 0 0 0 0 0.042649 0.076356 0.076356 0.076356 0.076356
  spline S319 degree 3 poles (62.6058, 40.8102) (62.6866, 40.7573) (62.8429, 40.6547) (62.9332, 40.4913) (62.9769, 40.4123) knots 0 0 0 0 0.028484 0.055146 0.055146 0.055146 0.055146
  spline S320 degree 3 poles (62.9769, 40.4123) (63.0078, 40.2852) (63.0904, 39.9452) (63.0867, 39.5944) (63.0843, 39.3747) knots 0 0 0 0 0.039108 0.104654 0.104654 0.104654 0.104654
  line L202 (63.0843, 39.3747) -> (63.0843, 36.3913)
  line L203 (63.0843, 36.3913) -> (63.7289, 36.3913)
  line L204 (63.7289, 36.3913) -> (63.7289, 35.7077)
  line L205 (63.7289, 35.7077) -> (63.0843, 35.7077)
  line L206 (63.0843, 35.7077) -> (63.0843, 34.4235)
  line L207 (63.0843, 34.4235) -> (62.2103, 33.8962)
  line L208 (62.2103, 33.8962) -> (62.2103, 35.7077)
  line L209 (62.2103, 35.7077) -> (61.3265, 35.7077)
  line L210 (61.3265, 35.7077) -> (61.3265, 36.3913)
  line L211 (61.3265, 36.3913) -> (62.2103, 36.3913)
  line L212 (62.2103, 36.3913) -> (62.2103, 39.4235)
  spline S321 degree 3 poles (62.2103, 39.4235) (62.2116, 39.5271) (62.2137, 39.6903) (62.1772, 39.8489) (62.1639, 39.9069) knots 0 0 0 0 0.030906 0.048705 0.048705 0.048705 0.048705
  spline S322 degree 3 poles (62.1639, 39.9069) (62.1458, 39.941) (62.1091, 40.0101) (62.045, 40.0551) (62.0126, 40.0778) knots 0 0 0 0 0.011413 0.023119 0.023119 0.023119 0.023119
  spline S323 degree 3 poles (62.0126, 40.0778) (61.9706, 40.0963) (61.8753, 40.1382) (61.7708, 40.1402) (61.7123, 40.1413) knots 0 0 0 0 0.013616 0.030961 0.030961 0.030961 0.030961
  spline S324 degree 3 poles (61.7123, 40.1413) (61.6556, 40.1393) (61.5265, 40.1347) (61.3984, 40.117) (61.3265, 40.1071) knots 0 0 0 0 0.016989 0.038747 0.038747 0.038747 0.038747
  line L213 (75.3451, 40.8932) -> (75.3451, 33.735)
  line L214 (75.3451, 33.735) -> (70.1693, 33.735)
  line L215 (70.1693, 33.735) -> (70.1693, 34.5798)
  line L216 (70.1693, 34.5798) -> (74.3978, 34.5798)
  line L217 (74.3978, 34.5798) -> (74.3978, 36.7721)
  line L218 (74.3978, 36.7721) -> (70.4379, 36.7721)
  line L219 (70.4379, 36.7721) -> (70.4379, 37.612)
  line L220 (70.4379, 37.612) -> (74.3978, 37.612)
  line L221 (74.3978, 37.612) -> (74.3978, 40.0485)
  line L222 (74.3978, 40.0485) -> (70.0033, 40.0485)
  line L223 (70.0033, 40.0485) -> (70.0033, 40.8932)
  line L224 (70.0033, 40.8932) -> (75.3451, 40.8932)
  line L225 (22.5695, 40.7129) -> (22.5695, 36.8237)
  line L226 (22.5695, 36.8237) -> (21.9762, 36.8237)
  line L227 (21.9762, 36.8237) -> (21.9762, 37.3767)
  spline S325 degree 3 poles (21.9762, 37.3767) (21.8156, 37.1898) (21.4896, 36.8104) (20.9912, 36.7609) (20.7384, 36.7358) knots 0 0 0 0 0.071082 0.144269 0.144269 0.144269 0.144269
  spline S326 degree 3 poles (20.7384, 36.7358) (20.6248, 36.7406) (20.4029, 36.7499) (20.194, 36.8253) (20.092, 36.8622) knots 0 0 0 0 0.033885 0.066204 0.066204 0.066204 0.066204
  spline S327 degree 3 poles (20.092, 36.8622) (20.0018, 36.9051) (19.832, 36.9859) (19.7086, 37.1274) (19.6508, 37.1936) knots 0 0 0 0 0.029622 0.055711 0.055711 0.055711 0.055711
  spline S328 degree 3 poles (19.6508, 37.1936) (19.6053, 37.2667) (19.5111, 37.418) (19.468, 37.5911) (19.4457, 37.6807) knots 0 0 0 0 0.025655 0.053138 0.053138 0.053138 0.053138
  spline S329 degree 3 poles (19.4457, 37.6807) (19.4351, 37.7645) (19.4083, 37.9771) (19.4088, 38.1916) (19.4091, 38.3215) knots 0 0 0 0 0.025326 0.064247 0.064247 0.064247 0.064247
  line L228 (19.4091, 38.3215) -> (19.4091, 40.7129)
  line L229 (19.4091, 40.7129) -> (20.0682, 40.7129)
  line L230 (20.0682, 40.7129) -> (20.0682, 38.3472)
  spline S330 degree 3 poles (20.0682, 38.3472) (20.0689, 38.229) (20.07, 38.0247) (20.1229, 37.8278) (20.1451, 37.7447) knots 0 0 0 0 0.035254 0.06095 0.06095 0.06095 0.06095
  spline S331 degree 3 poles (20.1451, 37.7447) (20.1763, 37.6812) (20.2399, 37.5517) (20.3579, 37.4685) (20.418, 37.4261) knots 0 0 0 0 0.020875 0.042549 0.042549 0.042549 0.042549
  spline S332 degree 3 poles (20.418, 37.4261) (20.4876, 37.3914) (20.6323, 37.3194) (20.7938, 37.3113) (20.8776, 37.3071) knots 0 0 0 0 0.023082 0.047934 0.047934 0.047934 0.047934
  spline S333 degree 3 poles (20.8776, 37.3071) (21.0126, 37.3178) (21.2801, 37.339) (21.4971, 37.4965) (21.6045, 37.5744) knots 0 0 0 0 0.039796 0.078805 0.078805 0.078805 0.078805
  spline S334 degree 3 poles (21.6045, 37.5744) (21.6931, 37.6994) (21.906, 37.9998) (21.9087, 38.3717) (21.9103, 38.5889) knots 0 0 0 0 0.045008 0.108186 0.108186 0.108186 0.108186
  line L231 (21.9103, 38.5889) -> (21.9103, 40.7129)
  line L232 (21.9103, 40.7129) -> (22.5695, 40.7129)
  line L233 (13.6522, 39.4604) -> (12.9711, 39.5447)
  spline S335 degree 3 poles (12.9711, 39.5447) (13.0337, 39.7305) (13.1548, 40.0901) (13.4334, 40.347) (13.568, 40.4712) knots 0 0 0 0 0.057776 0.111807 0.111807 0.111807 0.111807
  spline S336 degree 3 poles (13.568, 40.4712) (13.7292, 40.5672) (14.0715, 40.7711) (14.4703, 40.7905) (14.6813, 40.8008) knots 0 0 0 0 0.055438 0.117692 0.117692 0.117692 0.117692
  spline S337 degree 3 poles (14.6813, 40.8008) (14.9467, 40.7832) (15.4543, 40.7495) (15.8471, 40.4284) (16.0344, 40.2753) knots 0 0 0 0 0.077612 0.148419 0.148419 0.148419 0.148419
  spline S338 degree 3 poles (16.0344, 40.2753) (16.18, 40.0722) (16.4945, 39.6334) (16.5204, 39.092) (16.5343, 38.8013) knots 0 0 0 0 0.073419 0.158615 0.158615 0.158615 0.158615
  spline S339 degree 3 poles (16.5343, 38.8013) (16.5206, 38.5008) (16.4952, 37.9432) (16.1761, 37.4878) (16.0289, 37.2778) knots 0 0 0 0 0.088069 0.163473 0.163473 0.163473 0.163473
  spline S340 degree 3 poles (16.0289, 37.2778) (15.8449, 37.1198) (15.4679, 36.796) (14.9718, 36.7562) (14.7179, 36.7358) knots 0 0 0 0 0.070863 0.145168 0.145168 0.145168 0.145168
  spline S341 degree 3 poles (14.7179, 36.7358) (14.4716, 36.7561) (13.9888, 36.7958) (13.6228, 37.112) (13.4435, 37.2668) knots 0 0 0 0 0.072095 0.141285 0.141285 0.141285 0.141285
  spline S342 degree 3 poles (13.4435, 37.2668) (13.2995, 37.4728) (12.9872, 37.9195) (12.9624, 38.4663) (12.9491, 38.761) knots 0 0 0 0 0.073882 0.160281 0.160281 0.160281 0.160281
  spline S343 degree 3 poles (12.9491, 38.761) (12.9493, 38.7854) (12.9499, 38.844) (12.9517, 38.9026) (12.9528, 38.9368) knots 0 0 0 0 0.007325 0.017582 0.017582 0.017582 0.017582
  line L234 (12.9528, 38.9368) -> (15.8532, 38.9368)
  spline S344 degree 3 poles (15.8532, 38.9368) (15.8341, 39.132) (15.799, 39.4923) (15.5875, 39.7844) (15.4906, 39.9182) knots 0 0 0 0 0.057619 0.10631 0.10631 0.10631 0.10631
  spline S345 degree 3 poles (15.4906, 39.9182) (15.3745, 40.0175) (15.1402, 40.218) (14.8327, 40.2451) (14.6776, 40.2588) knots 0 0 0 0 0.044649 0.090131 0.090131 0.090131 0.090131
  spline S346 degree 3 poles (14.6776, 40.2588) (14.5628, 40.252) (14.3407, 40.2389) (14.1505, 40.1239) (14.0587, 40.0683) knots 0 0 0 0 0.033935 0.065626 0.065626 0.065626 0.065626
  spline S347 degree 3 poles (14.0587, 40.0683) (13.9759, 39.9902) (13.7946, 39.8191) (13.7024, 39.5867) (13.6522, 39.4604) knots 0 0 0 0 0.033751 0.073918 0.073918 0.073918 0.073918
  line L235 (5.4821, 40.7129) -> (5.4821, 36.8237)
  line L236 (5.4821, 36.8237) -> (4.8888, 36.8237)
  line L237 (4.8888, 36.8237) -> (4.8888, 37.4133)
  spline S348 degree 3 poles (4.8888, 37.4133) (4.8227, 37.2935) (4.7103, 37.0898) (4.5398, 36.9325) (4.4695, 36.8677) knots 0 0 0 0 0.040688 0.069205 0.069205 0.069205 0.069205
  spline S349 degree 3 poles (4.4695, 36.8677) (4.4039, 36.8292) (4.2731, 36.7525) (4.1219, 36.7414) (4.0465, 36.7358) knots 0 0 0 0 0.022479 0.044833 0.044833 0.044833 0.044833
  spline S350 degree 3 poles (4.0465, 36.7358) (3.9323, 36.7464) (3.6916, 36.7685) (3.4802, 36.8863) (3.369, 36.9482) knots 0 0 0 0 0.034017 0.071699 0.071699 0.071699 0.071699
  line L238 (3.369, 36.9482) -> (3.5961, 37.5598)
  spline S351 degree 3 poles (3.5961, 37.5598) (3.6749, 37.5182) (3.8266, 37.438) (3.9974, 37.4238) (4.0795, 37.417) knots 0 0 0 0 0.026437 0.050869 0.050869 0.050869 0.050869
  spline S352 degree 3 poles (4.0795, 37.417) (4.1497, 37.4224) (4.2899, 37.4332) (4.4084, 37.5091) (4.4677, 37.547) knots 0 0 0 0 0.020764 0.041509 0.041509 0.041509 0.041509
  spline S353 degree 3 poles (4.4677, 37.547) (4.5213, 37.5956) (4.6319, 37.6961) (4.6854, 37.8357) (4.713, 37.9077) knots 0 0 0 0 0.021403 0.044172 0.044172 0.044172 0.044172
  spline S354 degree 3 poles (4.713, 37.9077) (4.7451, 38.0297) (4.8112, 38.2818) (4.8189, 38.5423) (4.8229, 38.6767) knots 0 0 0 0 0.037715 0.077909 0.077909 0.077909 0.077909
  line L239 (4.8229, 38.6767) -> (4.8229, 40.7129)
  line L240 (4.8229, 40.7129) -> (5.4821, 40.7129)
  line L241 (2.9735, 40.7129) -> (2.9735, 36.8237)
  line L242 (2.9735, 36.8237) -> (2.3143, 36.8237)
  line L243 (2.3143, 36.8237) -> (2.3143, 40.7129)
  line L244 (2.3143, 40.7129) -> (2.9735, 40.7129)
  line L245 (1.5746, 39.552) -> (0.9227, 39.4494)
  spline S355 degree 3 poles (0.9227, 39.4494) (0.8987, 39.5703) (0.853, 39.7999) (0.6928, 39.9697) (0.6169, 40.05) knots 0 0 0 0 0.036133 0.068619 0.068619 0.068619 0.068619
  spline S356 degree 3 poles (0.6169, 40.05) (0.5194, 40.1108) (0.3056, 40.2439) (0.053, 40.2536) (-0.0843, 40.2588) knots 0 0 0 0 0.033906 0.074299 0.074299 0.074299 0.074299
  spline S357 degree 3 poles (-0.0843, 40.2588) (-0.2198, 40.2557) (-0.4611, 40.2501) (-0.6676, 40.1276) (-0.7582, 40.0738) knots 0 0 0 0 0.03982 0.070917 0.070917 0.070917 0.070917
  spline S358 degree 3 poles (-0.7582, 40.0738) (-0.8222, 40.0114) (-0.9453, 39.8913) (-0.9673, 39.7214) (-0.9779, 39.6399) knots 0 0 0 0 0.025989 0.049928 0.049928 0.049928 0.049928
  spline S359 degree 3 poles (-0.9779, 39.6399) (-0.9694, 39.5691) (-0.9523, 39.4259) (-0.8404, 39.3345) (-0.7838, 39.2883) knots 0 0 0 0 0.02054 0.041584 0.041584 0.041584 0.041584
  spline S360 degree 3 poles (-0.7838, 39.2883) (-0.7057, 39.2532) (-0.4891, 39.156) (-0.2578, 39.1004) (-0.11, 39.0649) knots 0 0 0 0 0.025642 0.071116 0.071116 0.071116 0.071116
  spline S361 degree 3 poles (-0.11, 39.0649) (0.0963, 39.0132) (0.4379, 38.9277) (0.7655, 38.7991) (0.8953, 38.7482) knots 0 0 0 0 0.063717 0.105491 0.105491 0.105491 0.105491
  spline S362 degree 3 poles (0.8953, 38.7482) (0.9822, 38.7006) (1.151, 38.6082) (1.2649, 38.4534) (1.3201, 38.3783) knots 0 0 0 0 0.029331 0.056937 0.056937 0.056937 0.056937
  spline S363 degree 3 poles (1.3201, 38.3783) (1.3623, 38.2971) (1.4473, 38.1334) (1.4589, 37.9493) (1.4647, 37.8564) knots 0 0 0 0 0.027121 0.054688 0.054688 0.054688 0.054688
  spline S364 degree 3 poles (1.4647, 37.8564) (1.4599, 37.7717) (1.4505, 37.6037) (1.3804, 37.4507) (1.3457, 37.3749) knots 0 0 0 0 0.025216 0.049996 0.049996 0.049996 0.049996
  spline S365 degree 3 poles (1.3457, 37.3749) (1.3024, 37.3041) (1.2158, 37.1626) (1.0864, 37.0588) (1.0216, 37.0068) knots 0 0 0 0 0.024672 0.049371 0.049371 0.049371 0.049371
  spline S366 degree 3 poles (1.0216, 37.0068) (0.9622, 36.9694) (0.831, 36.8869) (0.6832, 36.8401) (0.6023, 36.8146) knots 0 0 0 0 0.02098 0.046296 0.046296 0.046296 0.046296
  spline S367 degree 3 poles (0.6023, 36.8146) (0.5111, 36.7916) (0.3241, 36.7446) (0.1315, 36.7388) (0.0328, 36.7358) knots 0 0 0 0 0.028138 0.057638 0.057638 0.057638 0.057638
  spline S368 degree 3 poles (0.0328, 36.7358) (-0.1116, 36.74) (-0.3856, 36.748) (-0.6472, 36.8292) (-0.771, 36.8677) knots 0 0 0 0 0.04311 0.081794 0.081794 0.081794 0.081794
  spline S369 degree 3 poles (-0.771, 36.8677) (-0.8763, 36.9123) (-1.0723, 36.9953) (-1.2156, 37.1522) (-1.2819, 37.2247) knots 0 0 0 0 0.033843 0.06298 0.06298 0.06298 0.06298
  spline S370 degree 3 poles (-1.2819, 37.2247) (-1.3332, 37.3105) (-1.4449, 37.4974) (-1.4864, 37.7114) (-1.5089, 37.8271) knots 0 0 0 0 0.029774 0.064814 0.064814 0.064814 0.064814
  line L246 (-1.5089, 37.8271) -> (-0.8644, 37.915)
  spline S371 degree 3 poles (-0.8644, 37.915) (-0.844, 37.8214) (-0.8045, 37.6401) (-0.6733, 37.5095) (-0.6099, 37.4463) knots 0 0 0 0 0.02807 0.054357 0.054357 0.054357 0.054357
  spline S372 degree 3 poles (-0.6099, 37.4463) (-0.5272, 37.3973) (-0.3446, 37.2889) (-0.1315, 37.2817) (-0.0148, 37.2778) knots 0 0 0 0 0.028374 0.062736 0.062736 0.062736 0.062736
  spline S373 degree 3 poles (-0.0148, 37.2778) (0.1179, 37.2789) (0.3464, 37.2807) (0.5486, 37.3845) (0.6334, 37.428) knots 0 0 0 0 0.039091 0.067341 0.067341 0.067341 0.067341
  spline S374 degree 3 poles (0.6334, 37.428) (0.69, 37.478) (0.7969, 37.5726) (0.8177, 37.7133) (0.8275, 37.7795) knots 0 0 0 0 0.021851 0.041325 0.041325 0.041325 0.041325
  spline S375 degree 3 poles (0.8275, 37.7795) (0.8241, 37.8213) (0.8172, 37.9051) (0.7705, 37.9751) (0.747, 38.0102) knots 0 0 0 0 0.012342 0.0248 0.0248 0.0248 0.0248
  spline S376 degree 3 poles (0.747, 38.0102) (0.7141, 38.0449) (0.6423, 38.1209) (0.5464, 38.1631) (0.4943, 38.186) knots 0 0 0 0 0.014185 0.031058 0.031058 0.031058 0.031058
  spline S377 degree 3 poles (0.4943, 38.186) (0.4294, 38.2065) (0.2366, 38.2672) (0.0414, 38.3197) (-0.088, 38.3545) knots 0 0 0 0 0.020415 0.060621 0.060621 0.060621 0.060621
  spline S378 degree 3 poles (-0.088, 38.3545) (-0.2871, 38.4074) (-0.617, 38.495) (-0.9371, 38.6133) (-1.064, 38.6603) knots 0 0 0 0 0.061753 0.102322 0.102322 0.102322 0.102322
  spline S379 degree 3 poles (-1.064, 38.6603) (-1.1505, 38.7035) (-1.3198, 38.7882) (-1.4395, 38.9347) (-1.4979, 39.0063) knots 0 0 0 0 0.028671 0.05607 0.05607 0.05607 0.05607
  spline S380 degree 3 poles (-1.4979, 39.0063) (-1.5438, 39.0893) (-1.6407, 39.2645) (-1.6503, 39.4648) (-1.6554, 39.5703) knots 0 0 0 0 0.028058 0.059253 0.059253 0.059253 0.059253
  spline S381 degree 3 poles (-1.6554, 39.5703) (-1.6469, 39.6793) (-1.6297, 39.9006) (-1.5192, 40.0932) (-1.4631, 40.191) knots 0 0 0 0 0.032357 0.06571 0.06571 0.06571 0.06571
  spline S382 degree 3 poles (-1.4631, 40.191) (-1.39, 40.2834) (-1.2387, 40.4746) (-1.0209, 40.5846) (-0.9083, 40.6415) knots 0 0 0 0 0.0349 0.07223 0.07223 0.07223 0.07223
  spline S383 degree 3 poles (-0.9083, 40.6415) (-0.7808, 40.6879) (-0.516, 40.7844) (-0.2342, 40.7952) (-0.088, 40.8008) knots 0 0 0 0 0.04044 0.084019 0.084019 0.084019 0.084019
  spline S384 degree 3 poles (-0.088, 40.8008) (0.1404, 40.7943) (0.5528, 40.7827) (0.9086, 40.5774) (1.0674, 40.4858) knots 0 0 0 0 0.06725 0.121423 0.121423 0.121423 0.121423
  spline S385 degree 3 poles (1.0674, 40.4858) (1.1887, 40.3627) (1.4467, 40.101) (1.5303, 39.742) (1.5746, 39.552) knots 0 0 0 0 0.050868 0.10812 0.10812 0.10812 0.10812
  line L247 (2.9735, 36.1023) -> (2.9735, 35.3442)
  line L248 (2.9735, 35.3442) -> (2.3143, 35.3442)
  line L249 (2.3143, 35.3442) -> (2.3143, 36.1023)
  line L250 (2.3143, 36.1023) -> (2.9735, 36.1023)
  line L251 (9.6459, 42.2034) -> (9.6459, 36.8237)
  line L252 (9.6459, 36.8237) -> (9.0453, 36.8237)
  line L253 (9.0453, 36.8237) -> (9.0453, 37.3291)
  spline S386 degree 3 poles (9.0453, 37.3291) (8.9744, 37.2377) (8.8389, 37.0628) (8.6538, 36.9418) (8.5656, 36.8841) knots 0 0 0 0 0.034424 0.065839 0.065839 0.065839 0.065839
  spline S387 degree 3 poles (8.5656, 36.8841) (8.4684, 36.8409) (8.2624, 36.7492) (8.0367, 36.7405) (7.9174, 36.7358) knots 0 0 0 0 0.031594 0.067037 0.067037 0.067037 0.067037
  spline S388 degree 3 poles (7.9174, 36.7358) (7.7577, 36.7455) (7.4451, 36.7646) (7.172, 36.9174) (7.0385, 36.9922) knots 0 0 0 0 0.047311 0.092609 0.092609 0.092609 0.092609
  spline S389 degree 3 poles (7.0385, 36.9922) (6.9185, 37.0883) (6.6723, 37.2857) (6.5343, 37.5697) (6.4635, 37.7154) knots 0 0 0 0 0.045513 0.09343 0.09343 0.09343 0.09343
  spline S390 degree 3 poles (6.4635, 37.7154) (6.4069, 37.877) (6.2908, 38.2083) (6.2767, 38.5592) (6.2694, 38.739) knots 0 0 0 0 0.051054 0.104695 0.104695 0.104695 0.104695
  spline S391 degree 3 poles (6.2694, 38.739) (6.2771, 38.9301) (6.2919, 39.2999) (6.4212, 39.6464) (6.4836, 39.8138) knots 0 0 0 0 0.056969 0.110217 0.110217 0.110217 0.110217
  spline S392 degree 3 poles (6.4836, 39.8138) (6.5615, 39.9628) (6.7139, 40.2542) (6.9774, 40.4504) (7.1062, 40.5463) knots 0 0 0 0 0.049717 0.097233 0.097233 0.097233 0.097233
  spline S393 degree 3 poles (7.1062, 40.5463) (7.2427, 40.6205) (7.511, 40.7664) (7.8154, 40.7894) (7.965, 40.8008) knots 0 0 0 0 0.04603 0.090479 0.090479 0.090479 0.090479
  spline S394 degree 3 poles (7.965, 40.8008) (8.0707, 40.7956) (8.2766, 40.7857) (8.4649, 40.7022) (8.5564, 40.6616) knots 0 0 0 0 0.031458 0.061226 0.061226 0.061226 0.061226
  spline S395 degree 3 poles (8.5564, 40.6616) (8.6391, 40.613) (8.8008, 40.5181) (8.9257, 40.3783) (8.9867, 40.31) knots 0 0 0 0 0.028579 0.055867 0.055867 0.055867 0.055867
  line L254 (8.9867, 40.31) -> (8.9867, 42.2034)
  line L255 (8.9867, 42.2034) -> (9.6459, 42.2034)
  line L256 (2.1188, 53.7668) -> (-20.0663, 53.7668) construction
  line L257 (-20.0663, 53.7668) -> (-20.0663, 48.7668) construction
  line L258 (-20.0663, 48.7668) -> (2.1188, 48.7668) construction
  line L259 (2.1188, 48.7668) -> (2.1188, 53.7668) construction
  text T0 "Enterprise" font "Arial" height 5 align ink ink in box 0 x 0 at (2.1188, 53.7668) x (-1, 0) y (0, -1) spacing 1 height is em
  constraint perpendicular L256 L257
  constraint parallel L256 L258
  constraint parallel L257 L259
extrude "Extrude23" add sketch "Sketch24" along normal blind 2 text T0 bodies 15